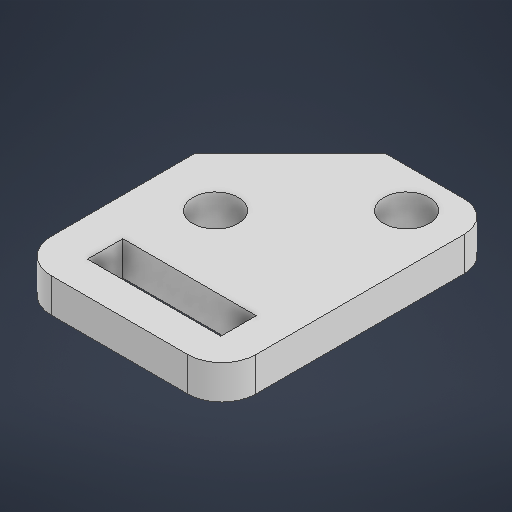
# Autodesk Inventor part: Hip
Saved by Autodesk Inventor 2026.2 (Build 302298010, 298A)
## iProperties
Created: 2026-05-07
Part Number: Hip
Material: Generic
Document SubType Name: Modeling
Designer: Martina
Density: 1 g/cm^3
Appearance: Default
Author: Martina
Autodesk Inventor part; units mm, degrees
ref_plane "YZ Plane" through (0, 0, 0) normal (1, 0, 0) x (0, 1, 0)
ref_plane "XZ Plane" through (0, 0, 0) normal (0, 1, 0) x (-1, 0, 0)
ref_plane "XY Plane" through (0, 0, 0) normal (0, 0, 1) x (1, 0, 0)
sketch "Sketch1" plane through (0, 0, 0) normal (0, 1, 0) x (-1, 0, 0)
  line L0 (9, 0) -> (45, 0)
  line L1 (54, -9) -> (54, -46.8)
  line L2 (28.8, -72) -> (8.1, -72)
  line L3 (0, -63.9) -> (0, -9)
  arc A0 (54, -9) -> (45, 0) centre (45, -9) ccw
  arc A1 (9, 0) -> (0, -9) centre (9, -9) ccw
  arc A2 (0, -63.9) -> (8.1, -72) centre (8.1, -63.9) ccw
  line L4 (54, -46.8) -> (28.8, -72)
  circle A3 centre (38.233, -36.5794) radius 6
  circle A4 centre (13.039, -61.766) radius 6
  line L5 (44.015, -8.55) -> (8.815, -8.55)
  line L6 (8.815, -8.55) -> (8.815, -17.9)
  line L7 (8.815, -17.9) -> (44.015, -17.9)
  line L8 (44.015, -17.9) -> (44.015, -8.55)
  point P0 (0, 0)
  point P1 (54, -72)
  point P2 (54, 0)
  point P3 (0, -72)
  dimension "d2" = 9
  dimension "d3" = 8.1
  dimension "d7" = 20.7
  dimension "d8" = 36
  dimension "d9" = 37.8
  dimension "d10" = 9
  dimension "d11" = 54.9
  dimension "d12" = 12
  dimension "d13" = 12
  dimension "d14" = 15.767
  dimension "d15" = 18.376
  dimension "d16" = 10.234
  dimension "d17" = 13.039
  dimension "d18" = 38.233
  dimension "d19" = 9.35
  dimension "d20" = 35.2
  dimension "d21" = 8.55
  dimension "d22" = 8.815
  dimension "d23" = 9.985
  dimension "d26" = 23.6245
  constraints: 18 end point, 8 point on line, 6 point on circle, 6 tangent, 5 centre point, 4 parallel, 2 horizontal, 2 perpendicular, 1 equal radius
  measures "d2" radius of A0
  measures "d3" radius of A2
  measures "d7" distance of L2.start L2.end
  measures "d8" distance of L0.start L0.end
  measures "d9" distance of L1.start L1.end
  measures "d10" radius of A1
  measures "d11" distance of L3.start L3.end
  measures "d12" diameter of A3
  measures "d13" diameter of A4
  measures "d14" distance from line of A3.centre L1
  measures "d15" distance from line of L4 A3.centre
  measures "d16" distance from line of L2 A4.centre
  measures "d17" distance from line of L3 A4.centre
  measures "d18" distance from line of L3 A3.centre
  measures "d19" distance of L7.end L5.start
  measures "d20" distance of L6.end L7.end
  measures "d21" distance between parallel lines of L5 L0
  measures "d22" distance between parallel lines of L3 L6
  measures "d23" distance between parallel lines of L8 L1
extrude "Extrusion1" add sketch "Sketch1" along normal blind 9
body "Solid1"
